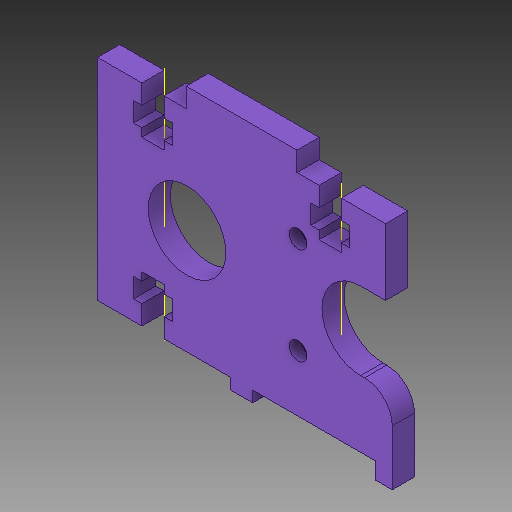
# Autodesk Inventor part: Motorhalter_links
Saved by Autodesk Inventor 2019 (Build 230136000, 136)
## iProperties
Created: 2022-10-31
Part Number: Motorhalter_links
Material: Generisch
Document SubType Name: Modeling
Designer: RP
Density: 1 g/cm^3
Appearance: Violett
Author: RP
Autodesk Inventor part; units mm, degrees
ref_plane "YZ Plane" through (0, 0, 0) normal (1, 0, 0) x (0, 1, 0)
ref_plane "XZ Plane" through (0, 0, 0) normal (0, 1, 0) x (-1, 0, 0)
ref_plane "XY Plane" through (0, 0, 0) normal (0, 0, 1) x (1, 0, 0)
sketch "Skizze1" plane through (0, 0, 0) normal (0, 0, 1) x (1, 0, 0)
  circle A0 centre (-60.768, 178.1277) radius 7
  circle A1 centre (-40.718, 169.3777) radius 1.6
  circle A2 centre (-40.718, 186.8777) radius 1.6
  line L0 (-23.718, 156.1277) -> (-23.718, 166.1277)
  arc A3 (-23.718, 166.1277) -> (-28.718, 171.1277) centre (-28.718, 166.1277) ccw
  line L1 (-28.718, 171.1277) -> (-29.418, 171.1277)
  arc A4 (-29.418, 185.1277) -> (-29.418, 171.1277) centre (-29.418, 178.1277) ccw
  line L2 (-40.918, 197.1277) -> (-40.918, 200.6277)
  line L3 (-40.918, 200.6277) -> (-60.918, 200.6277)
  line L4 (-68.918, 197.1277) -> (-76.918, 197.1277)
  line L5 (-76.918, 197.1277) -> (-76.918, 159.1277)
  line L6 (-76.918, 159.1277) -> (-68.918, 159.1277)
  line L7 (-64.918, 159.1277) -> (-26.718, 159.1277)
  line L8 (-26.718, 159.1277) -> (-26.718, 156.1277)
  line L9 (-26.718, 156.1277) -> (-23.718, 156.1277)
  line L10 (-36.5327, 178.1277) -> (-67.768, 178.1277) construction
  line L11 (-40.718, 169.3777) -> (-40.718, 186.8777) construction
  line L12 (-32.918, 197.1277) -> (-32.918, 193.6277)
  line L13 (-32.918, 193.6277) -> (-31.418, 193.6277)
  line L14 (-31.418, 193.6277) -> (-31.418, 190.1277)
  line L15 (-31.418, 190.1277) -> (-32.918, 190.1277)
  line L16 (-32.918, 190.1277) -> (-32.918, 188.6277)
  line L17 (-32.918, 188.6277) -> (-36.918, 188.6277)
  line L18 (-36.918, 188.6277) -> (-36.918, 190.1277)
  line L19 (-36.918, 190.1277) -> (-38.418, 190.1277)
  line L20 (-38.418, 190.1277) -> (-38.418, 193.6277)
  line L21 (-38.418, 193.6277) -> (-36.918, 193.6277)
  line L22 (-36.918, 197.1277) -> (-36.918, 193.6277)
  line L23 (-34.918, 197.9429) -> (-34.918, 190.1833) construction
  line L24 (-32.918, 197.1277) -> (-24.918, 197.1277)
  line L25 (-50.918, 190.3199) -> (-50.918, 199.5586) construction
  line L26 (-68.918, 190.1277) -> (-68.918, 188.6277)
  line L27 (-66.918, 197.9429) -> (-66.918, 190.1833) construction
  line L28 (-64.918, 197.1277) -> (-64.918, 193.6277)
  line L29 (-68.918, 188.6277) -> (-64.918, 188.6277)
  line L30 (-63.418, 193.6277) -> (-64.918, 193.6277)
  line L31 (-63.418, 190.1277) -> (-63.418, 193.6277)
  line L32 (-64.918, 188.6277) -> (-64.918, 190.1277)
  line L33 (-64.918, 190.1277) -> (-63.418, 190.1277)
  line L34 (-70.418, 190.1277) -> (-68.918, 190.1277)
  line L35 (-68.918, 193.6277) -> (-70.418, 193.6277)
  line L36 (-70.418, 193.6277) -> (-70.418, 190.1277)
  line L37 (-68.918, 197.1277) -> (-68.918, 193.6277)
  line L38 (-29.418, 185.1277) -> (-24.918, 185.1277)
  line L39 (-24.918, 185.1277) -> (-24.918, 197.1277)
  line L40 (-60.918, 200.6277) -> (-60.918, 197.1277)
  line L41 (-36.918, 197.1277) -> (-40.918, 197.1277)
  line L42 (-60.918, 197.1277) -> (-64.918, 197.1277)
  line L43 (-68.918, 162.6277) -> (-70.418, 162.6277)
  line L44 (-70.418, 162.6277) -> (-70.418, 166.1277)
  line L45 (-70.418, 166.1277) -> (-68.918, 166.1277)
  line L46 (-68.918, 166.1277) -> (-68.918, 167.6277)
  line L47 (-68.918, 167.6277) -> (-64.918, 167.6277)
  line L48 (-64.918, 167.6277) -> (-64.918, 166.1277)
  line L49 (-64.918, 166.1277) -> (-63.418, 166.1277)
  line L50 (-63.418, 166.1277) -> (-63.418, 162.6277)
  line L51 (-63.418, 162.6277) -> (-64.918, 162.6277)
  line L52 (-64.918, 159.1277) -> (-64.918, 162.6277)
  line L53 (-68.918, 159.1277) -> (-68.918, 162.6277)
  circle A5 centre (-49.518, 178.1277) radius 1.95
  point P0 (0, 0)
  point P1 (-56.218, 159.1277)
  point P2 (-36.918, 159.1277)
  point P3 (-40.718, 178.1277)
  dimension "d51" = 14
  dimension "d4" = 14
  dimension "d5" = 3
  dimension "d7" = 5
  dimension "d8" = 7
  dimension "d9" = 4.3
  dimension "d27" = 32
  dimension "d28" = 10
  dimension "d31" = 10
  dimension "d33" = 20
  dimension "d34" = 3.5
  dimension "d37" = 4
  dimension "d38" = 7
  dimension "d39" = 3.5
  dimension "d40" = 3.5
  dimension "d41" = 1.5
  dimension "d42" = 5.8
  dimension "d43" = 22.5
  dimension "d45" = 3
  dimension "d49" = 11.25
  dimension "d50" = 3.9
  constraints: 108 end point, 27 point on line, 14 symmetric about line, 13 collinear, 5 centre point, 5 perpendicular, 5 point on circle, 5 vertical, 4 tangent, 3 horizontal, 1 horizontal alignment, 1 midpoint, 1 parallel, 8 other
  measures "d4" distance between parallel lines of L8 L11
  measures "d5" distance of L8.end L0.start
  measures "d7" radius of A3
  measures "d8" distance between parallel lines of L1 L10
  measures "d9" distance edge to line of A4 L11
  measures "d27" distance between parallel lines of L27 L23
  measures "d28" distance between parallel lines of L39 L23
  measures "d31" distance between parallel lines of L27 L5
  measures "d33" distance of L2.end L3.end
  measures "d34" distance of L3.end L40.end
  measures "d37" distance between parallel lines of L22 L12
  measures "d38" distance between parallel lines of L14 L20
  measures "d39" distance of L12.start L13.start
  measures "d40" distance of L13.end L15.start
  measures "d41" distance of L16.start L16.end
  measures "d42" distance between parallel lines of L23 L11
  measures "d43" distance between parallel lines of L3 L10
  measures "d45" distance of L7.end L8.end
  measures "d49" distance of point (-60.768, 178.128) A5.centre
  measures "d50" diameter of A5
extrude "Extrusion1" add sketch "Skizze1" along normal mid plane 4 contours L9 L8 L7 L52 L51 L50 L49 L48 L47 L46 L45 L44 L43 L53 L6 L5 L4 L37 L35 L36 L34 L26 L29 L32 L33 L31 L30 L28 L42 L40 L3 L2 L41 L22 L21 L20 L19 L18 L17 L16 L15 L14 L13 L12 L24 L39 L38 A4 L1 A3 L0 | A5
sketch "Skizze2" plane through (0, 0, -2) normal (0, 0, -1) x (-1, 0, 0)
  circle A0 centre (60.768, 178.1277) radius 7 projected
  circle A1 centre (40.718, 186.8777) radius 1.6 projected
  circle A2 centre (40.718, 169.3777) radius 1.6 projected
  line L0 (23.718, 166.1277) -> (23.718, 156.1277) projected
  line L1 (23.718, 156.1277) -> (26.718, 156.1277) projected
  line L2 (26.718, 156.1277) -> (26.718, 159.1277) projected
  line L3 (26.718, 159.1277) -> (64.918, 159.1277) projected
  line L4 (64.918, 159.1277) -> (64.918, 162.6277) projected
  line L5 (64.918, 162.6277) -> (63.418, 162.6277) projected
  line L6 (63.418, 162.6277) -> (63.418, 166.1277) projected
  line L7 (63.418, 166.1277) -> (64.918, 166.1277) projected
  line L8 (64.918, 166.1277) -> (64.918, 167.6277) projected
  line L9 (64.918, 167.6277) -> (68.918, 167.6277) projected
  line L10 (68.918, 167.6277) -> (68.918, 166.1277) projected
  line L11 (68.918, 166.1277) -> (70.418, 166.1277) projected
  line L12 (70.418, 166.1277) -> (70.418, 162.6277) projected
  line L13 (70.418, 162.6277) -> (68.918, 162.6277) projected
  line L14 (68.918, 162.6277) -> (68.918, 159.1277) projected
  line L15 (68.918, 159.1277) -> (76.918, 159.1277) projected
  line L16 (76.918, 159.1277) -> (76.918, 197.1277) projected
  line L17 (76.918, 197.1277) -> (68.918, 197.1277) projected
  line L18 (68.918, 197.1277) -> (68.918, 193.6277) projected
  line L19 (68.918, 193.6277) -> (70.418, 193.6277) projected
  line L20 (70.418, 193.6277) -> (70.418, 190.1277) projected
  line L21 (70.418, 190.1277) -> (68.918, 190.1277) projected
  line L22 (68.918, 190.1277) -> (68.918, 188.6277) projected
  line L23 (68.918, 188.6277) -> (64.918, 188.6277) projected
  line L24 (64.918, 188.6277) -> (64.918, 190.1277) projected
  line L25 (64.918, 190.1277) -> (63.418, 190.1277) projected
  line L26 (63.418, 190.1277) -> (63.418, 193.6277) projected
  line L27 (63.418, 193.6277) -> (64.918, 193.6277) projected
  line L28 (64.918, 193.6277) -> (64.918, 197.1277) projected
  line L29 (64.918, 197.1277) -> (60.918, 197.1277) projected
  line L30 (60.918, 197.1277) -> (60.918, 200.6277) projected
  line L31 (60.918, 200.6277) -> (40.918, 200.6277) projected
  line L32 (40.918, 200.6277) -> (40.918, 197.1277) projected
  line L33 (40.918, 197.1277) -> (36.918, 197.1277) projected
  line L34 (36.918, 197.1277) -> (36.918, 193.6277) projected
  line L35 (36.918, 193.6277) -> (38.418, 193.6277) projected
  line L36 (38.418, 193.6277) -> (38.418, 190.1277) projected
  line L37 (38.418, 190.1277) -> (36.918, 190.1277) projected
  line L38 (36.918, 190.1277) -> (36.918, 188.6277) projected
  line L39 (36.918, 188.6277) -> (32.918, 188.6277) projected
  line L40 (32.918, 188.6277) -> (32.918, 190.1277) projected
  line L41 (32.918, 190.1277) -> (31.418, 190.1277) projected
  line L42 (31.418, 190.1277) -> (31.418, 193.6277) projected
  line L43 (31.418, 193.6277) -> (32.918, 193.6277) projected
  line L44 (32.918, 193.6277) -> (32.918, 197.1277) projected
  line L45 (32.918, 197.1277) -> (24.918, 197.1277) projected
  line L46 (24.918, 197.1277) -> (24.918, 185.1277) projected
  line L47 (24.918, 185.1277) -> (29.418, 185.1277) projected
  arc A3 (29.418, 171.1277) -> (29.418, 185.1277) centre (29.418, 178.1277) ccw projected
  line L48 (29.418, 171.1277) -> (28.718, 171.1277) projected
  arc A4 (28.718, 171.1277) -> (23.718, 166.1277) centre (28.718, 166.1277) ccw projected
  circle A5 centre (40.718, 169.3777) radius 1.6 projected
  line L49 (42.9634, 171.623) -> (43.7853, 168.5558)
  line L50 (43.7853, 168.5558) -> (41.5399, 166.3104)
  line L51 (41.5399, 166.3104) -> (38.4727, 167.1323)
  line L52 (38.4727, 167.1323) -> (37.6508, 170.1995)
  line L53 (37.6508, 170.1995) -> (39.8962, 172.4449)
  line L54 (39.8962, 172.4449) -> (42.9634, 171.623)
  line L55 (42.9634, 189.123) -> (43.7853, 186.0558)
  line L56 (43.7853, 186.0558) -> (41.5399, 183.8104)
  line L57 (41.5399, 183.8104) -> (38.4727, 184.6323)
  line L58 (38.4727, 184.6323) -> (37.6508, 187.6995)
  line L59 (37.6508, 187.6995) -> (39.8962, 189.9449)
  line L60 (39.8962, 189.9449) -> (42.9634, 189.123)
  line L61 (38.418, 190.1277) -> (36.918, 188.6277) construction
  point P0 (0, 0)
  dimension "d52" = 5.5
  constraints: 26 end point, 2 coincident, 2 parallel, 1 equal length, 26 other
  measures "d52" distance between parallel lines of L50 L53
extrude "Extrusion2" cut sketch "Skizze2" against normal blind 2 contours L49 L50 L51 L52 L53 L54 | L55 L56 L57 L58 L59 L60
sketch "Skizze3" plane through (-64.918, 159.1277, 2) normal (0, -1, 0) x (1, 0, 0)
  line L0 (0, 0) -> (38.2, 0) projected
  line L1 (12, -4) -> (16, -4)
  line L2 (16, -4) -> (16, 0)
  line L3 (16, 0) -> (12, 0)
  line L4 (12, 0) -> (12, -4)
  line L5 (-12, -4) -> (-12, 0) projected
  point P0 (64.918, -2)
  point P1 (-2, -2)
  dimension "d55" = 4
  dimension "d57" = 24
  constraints: 8 end point, 2 parallel, 2 point on line, 1 horizontal, 1 perpendicular
  measures "d55" distance between parallel lines of L2 L4
  measures "d57" distance between parallel lines of L4 L5
extrude "Extrusion3" add sketch "Skizze3" along normal blind 2
